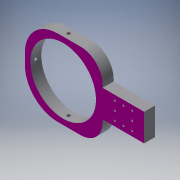
# Autodesk Inventor part: rotation-recuperation
Saved by Autodesk Inventor 2017 (Build 210142000, 142)
## iProperties
Created: 2018-04-01
Part Number: rotation-recuperation
Material: Generic
Document SubType Name: Modeling
Designer: franc
Density: 1 g/cm^3
Appearance: Default
Author: franc
Autodesk Inventor part; units mm, degrees
ref_plane "YZ Plane" through (0, 0, 0) normal (1, 0, 0) x (0, 1, 0)
ref_plane "XZ Plane" through (0, 0, 0) normal (0, 1, 0) x (-1, 0, 0)
ref_plane "XY Plane" through (0, 0, 0) normal (0, 0, 1) x (1, 0, 0)
sketch "Esquisse1" plane through (0, 0, 0) normal (0, 1, 0) x (-1, 0, 0)
  line L0 (-17.8264, 13.8129) -> (-17.8264, 6.3115) projected
  line L1 (20.1692, 13.8129) -> (-17.8264, 13.8129) projected
  line L2 (20.1692, 6.3115) -> (20.1692, 13.8129) projected
  line L3 (20.1692, 6.3115) -> (20.1692, 5.0615) projected
  arc A0 (19.9192, 4.8115) -> (20.1692, 5.0615) centre (19.9192, 5.0615) ccw projected
  line L4 (16.2667, 4.8115) -> (19.9192, 4.8115) projected
  arc A1 (16.2667, 4.8115) -> (16.0167, 4.5615) centre (16.2667, 4.5615) ccw projected
  line L5 (16.0167, -1.9385) -> (16.0167, 4.5615) projected
  arc A2 (16.0167, -1.9385) -> (16.2667, -2.1885) centre (16.2667, -1.9385) ccw projected
  line L6 (18.6692, -2.1885) -> (16.2667, -2.1885) projected
  arc A3 (18.6692, -2.1885) -> (18.9192, -1.9385) centre (18.6692, -1.9385) ccw projected
  line L7 (18.9192, 2.8115) -> (18.9192, -1.9385) projected
  arc A4 (18.9192, 3.8115) -> (18.9192, 2.8115) centre (18.9192, 3.3115) ccw projected
  line L8 (19.9192, 3.8115) -> (18.9192, 3.8115) projected
  arc A5 (20.1692, 3.5615) -> (19.9192, 3.8115) centre (19.9192, 3.5615) ccw projected
  line L9 (20.1692, 3.5615) -> (20.1692, -3.6892) projected
  line L10 (20.1692, -11.1878) -> (20.1692, -3.6892) projected
  line L11 (20.1692, -11.1878) -> (-17.8264, -11.1878) projected
  line L12 (-17.8264, -3.6892) -> (-17.8264, -11.1878) projected
  line L13 (-17.8264, 3.5615) -> (-17.8264, -3.6892) projected
  arc A6 (-17.5764, 3.8115) -> (-17.8264, 3.5615) centre (-17.5764, 3.5615) ccw projected
  line L14 (-16.5764, 3.8115) -> (-17.5764, 3.8115) projected
  arc A7 (-16.5764, 2.8115) -> (-16.5764, 3.8115) centre (-16.5764, 3.3115) ccw projected
  line L15 (-16.5764, -1.9385) -> (-16.5764, 2.8115) projected
  arc A8 (-16.5764, -1.9385) -> (-16.3264, -2.1885) centre (-16.3264, -1.9385) ccw projected
  line L16 (-13.9239, -2.1885) -> (-16.3264, -2.1885) projected
  arc A9 (-13.9239, -2.1885) -> (-13.6739, -1.9385) centre (-13.9239, -1.9385) ccw projected
  line L17 (-13.6739, 4.5615) -> (-13.6739, -1.9385) projected
  arc A10 (-13.6739, 4.5615) -> (-13.9239, 4.8115) centre (-13.9239, 4.5615) ccw projected
  line L18 (-17.5764, 4.8115) -> (-13.9239, 4.8115) projected
  arc A11 (-17.8264, 5.0615) -> (-17.5764, 4.8115) centre (-17.5764, 5.0615) ccw projected
  line L19 (-17.8264, 6.3115) -> (-17.8264, 5.0615) projected
  circle A12 centre (-14.8286, -6.6881) radius 1 projected
  circle A13 centre (-14.8286, 9.3119) radius 1 projected
  circle A14 centre (17.1714, 9.3119) radius 1 projected
  circle A15 centre (17.1714, -6.6881) radius 1 projected
  circle A16 centre (-6.8286, -6.6881) radius 1 projected
  circle A17 centre (-6.8286, 9.3119) radius 1 projected
  circle A18 centre (9.1714, 9.3119) radius 1 projected
  circle A19 centre (9.1714, -6.6881) radius 1 projected
  circle A20 centre (-6.8286, 1.3119) radius 1 projected
  circle A21 centre (1.1714, 9.3119) radius 1 projected
  circle A22 centre (9.1714, 1.3119) radius 1 projected
  circle A23 centre (1.1714, -6.6881) radius 1 projected
  line L20 (6.1717, 4.2695) -> (6.1717, -1.6458) projected
  line L21 (3.8644, 4.2695) -> (6.1717, 4.2695) projected
  arc A24 (3.8644, 4.2695) -> (-1.5216, 4.2695) centre (1.1714, 1.3119) ccw projected
  line L22 (-3.8289, 4.2695) -> (-1.5216, 4.2695) projected
  line L23 (-3.8289, -1.6458) -> (-3.8289, 4.2695) projected
  line L24 (-1.5216, -1.6458) -> (-3.8289, -1.6458) projected
  arc A25 (-1.5216, -1.6458) -> (3.8644, -1.6458) centre (1.1714, 1.3119) ccw projected
  line L25 (6.1717, -1.6458) -> (3.8644, -1.6458) projected
  line L26 (-17.8264, 13.8129) -> (20.1692, 13.8129)
  line L27 (20.1692, 13.8129) -> (20.1692, -11.1878)
  line L28 (20.1692, -11.1878) -> (-17.8264, -11.1878)
  line L29 (-17.8264, -11.1878) -> (-17.8264, 13.8129)
  circle A26 centre (-6.8286, -6.6881) radius 1
  circle A27 centre (-6.8286, 1.3119) radius 1
  circle A28 centre (-6.8286, 9.3119) radius 1
  circle A29 centre (1.1714, 9.3119) radius 1
  circle A30 centre (1.1714, -6.6881) radius 1
  circle A31 centre (9.1714, -6.6881) radius 1
  circle A32 centre (9.1714, 1.3119) radius 1
  circle A33 centre (9.1714, 9.3119) radius 1
  constraints: 8 centre point, 8 coincident, 8 concentric, 8 end point, 2 parallel, 1 horizontal, 1 perpendicular
extrude "Extrusion1" add sketch "Esquisse1" along normal blind 10 contours L1 L2 L3 A0 L4 A1 L5 A2 L6 A3 L7 A4 L8 A5 L9 L10 L11 L12 L13 A6 L14 A7 L15 A8 L16 A9 L17 A10 L18 A11 L19 L0 | A11 L18 A10 L17 A9 L16 A8 L15 A7 L14 A6 L29 | L27 A5 L8 A4 L7 A3 L6 A2 L5 A1 L4 A0 | A12 | A13 | A14 | A15 | L20 L25 A25 L24 L23 L22 A24 L21
sketch "Esquisse2" plane through (0, 0, 0) normal (0, -1, 0) x (1, 0, 0)
  circle A0 centre (-56.1714, 1.3122) radius 30 projected
  line L0 (-61.1714, 36.3122) -> (-40.1692, 36.3122)
  line L1 (-20.1692, 16.3122) -> (-20.1692, -13.6878)
  line L2 (-40.1692, -33.6878) -> (-61.1714, -33.6878)
  line L3 (-91.1714, -3.6878) -> (-91.1714, 6.3122)
  arc A1 (-61.1714, 36.3122) -> (-91.1714, 6.3122) centre (-61.1714, 6.3122) ccw
  arc A2 (-91.1714, -3.6878) -> (-61.1714, -33.6878) centre (-61.1714, -3.6878) ccw
  line L4 (-20.1692, -11.1878) -> (-20.1692, 13.8129) projected
  arc A3 (-20.1692, 16.3122) -> (-40.1692, 36.3122) centre (-40.1692, 16.3122) ccw
  arc A4 (-40.1692, -33.6878) -> (-20.1692, -13.6878) centre (-40.1692, -13.6878) ccw
  point P0 (0, 0)
  dimension "d4" = 35
  dimension "d5" = 35
  dimension "d6" = 35
  dimension "d7" = 30
  dimension "d8" = 30
  dimension "d9" = 0
  dimension "d10" = 20
  dimension "d11" = 20
  constraints: 8 end point, 8 point on circle, 8 tangent, 4 centre point, 2 parallel, 1 horizontal, 1 perpendicular
  measures "d4" distance from line of L2 A0.centre
  measures "d5" distance from line of L0 A0.centre
  measures "d6" distance from line of L3 A0.centre
  measures "d7" radius of A1
  measures "d8" radius of A2
  measures "d9" distance between parallel lines of L4 L1
  measures "d10" radius of A3
  measures "d11" radius of A4
extrude "Extrusion2" add sketch "Esquisse2" against normal blind 10
sketch "Esquisse3" plane through (-61.1714, 0, 36.3122) normal (0, 0, 1) x (1, 0, 0)
  line L0 (35, 92.5) -> (35, -82.5)
  circle A0 centre (5, 5) radius 1.5
  line L1 (0, 10) -> (21.0022, 10) projected
  point P0 (61.1714, 0)
  dimension "d14" = 30
  dimension "d15" = 3
  dimension "d16" = 5
  constraints: 2 end point, 1 centre point, 1 vertical, 2 other
  measures "d14" distance from line of A0.centre L0
  measures "d15" diameter of A0
  measures "d16" distance from line of L1 A0.centre
extrude "Extrusion3" cut sketch "Esquisse3" against normal through all
sketch "Esquisse4" plane through (-91.1714, 0, -3.6878) normal (-1, 0, 0) x (0, 0, 1)
  line L0 (35, 92.5) -> (35, -82.5)
  circle A0 centre (5, 5) radius 1.5
  line L1 (0, 0) -> (10, 0) projected
  point P0 (3.6878, 0)
  dimension "d19" = 3
  dimension "d20" = 30
  dimension "d21" = 5
  constraints: 2 end point, 1 centre point, 1 vertical, 2 other
  measures "d19" diameter of A0
  measures "d20" distance from line of L0 A0.centre
  measures "d21" distance from line of L1 A0.centre
extrude "Extrusion4" cut sketch "Esquisse4" against normal up to next
